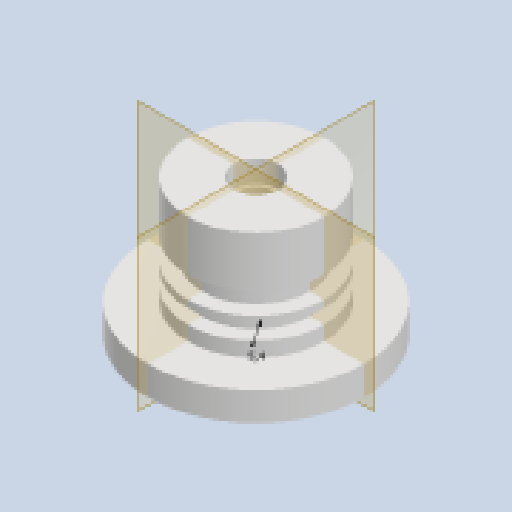
# Autodesk Inventor part: диск
Saved by Autodesk Inventor 2024.2 (Build 282272000, 272)
## iProperties
Created: 2025-11-25
Part Number: диск
Material: Типовые
Document SubType Name: Modeling
Designer: katya_notebook
Density: 1 g/cm^3
Appearance: По умолчанию
Author: katya_notebook
Autodesk Inventor part; units mm, degrees
ref_plane "XZ Plane" through (0, 0, 0) normal (0, 1, 0) x (-1, 0, 0)
sketch "Эскиз1" plane through (0, 0, 0) normal (0, 1, 0) x (-1, 0, 0)
  circle A0 centre (0, 0) radius 9.5
  dimension "d0" = 19
  constraints: 1 centre point, 1 coincident
  measures "d0" diameter of A0
extrude "Выдавливание1" add sketch "Эскиз1" along normal blind 5
sketch "Эскиз2" plane through (0, 0, 0) normal (0, -1, 0) x (1, 0, 0)
  circle A0 centre (0, 0) radius 7.5
  dimension "d3" = 15
  constraints: 1 centre point, 1 coincident
  measures "d3" diameter of A0
extrude "Выдавливание2" add sketch "Эскиз2" along normal blind 3
sketch "Эскиз3" plane through (0, -3, 0) normal (0, -1, 0) x (1, 0, 0)
  circle A0 centre (0, 0) radius 9.5
  dimension "d15" = 19
  constraints: 1 centre point, 1 coincident
  measures "d15" diameter of A0
extrude "Выдавливание3" add sketch "Эскиз3" along normal blind 1
sketch "Эскиз4" plane through (0, -4, 0) normal (0, -1, 0) x (1, 0, 0)
  circle A0 centre (0, 0) radius 7.5
  dimension "d17" = 15
  constraints: 1 centre point, 1 coincident
  measures "d17" diameter of A0
extrude "Выдавливание4" add sketch "Эскиз4" along normal blind 2
sketch "Эскиз5" plane through (0, -6, 0) normal (0, -1, 0) x (1, 0, 0)
  circle A0 centre (0, 0) radius 9.5
  dimension "d16" = 19
  constraints: 1 centre point, 1 coincident
  measures "d16" diameter of A0
extrude "Выдавливание5" add sketch "Эскиз5" along normal blind 2
sketch "Эскиз8" plane through (0, -8, 0) normal (0, -1, 0) x (1, 0, 0)
  circle A0 centre (0, 0) radius 15
  dimension "d21" = 30
  constraints: 1 centre point, 1 coincident
  measures "d21" diameter of A0
extrude "Выдавливание8" add sketch "Эскиз8" along normal blind 2
sketch "Эскиз6" plane through (0, 5, 0) normal (0, 1, 0) x (1, 0, 0)
  circle A0 centre (0, 0) radius 2.6
  dimension "d12" = 5.2
  constraints: 1 centre point, 1 coincident
  measures "d12" diameter of A0
extrude "Выдавливание6" cut sketch "Эскиз6" against normal blind 27
sketch "Эскиз10" plane through (0, -10, 0) normal (0, -1, 0) x (1, 0, 0)
  circle A0 centre (0, 0) radius 15 projected
  circle A1 centre (0, 0) radius 15
  circle A2 centre (0, 0) radius 2.5 projected
  circle A3 centre (0, 0) radius 2.5
  constraints: 2 centre point, 2 coincident, 2 concentric
ref_plane "РабПлоскость1" through (-11.6426, -12, -11.6426) normal (0, -1, 0) x (1, 0, 0)
extrude "Выдавливание10" add sketch "Эскиз10" along normal up to surface (2 mm away)
sketch "Эскиз11" plane through (0, -12, 0) normal (0, -1, 0) x (1, 0, 0)
  circle A0 centre (0, 0) radius 5 projected
  circle A1 centre (0, 0) radius 5
  circle A2 centre (0, 0) radius 2.7
  point P0 (0, 0)
  dimension "d38" = 5.4
  constraints: 2 centre point, 1 concentric
  measures "d38" diameter of A2
ref_plane "РабПлоскость2" through (-5.2921, -22, -5.2921) normal (0, -1, 0) x (1, 0, 0)
sketch "Эскиз13" plane through (0, 5, 0) normal (0, 1, 0) x (1, 0, 0)
  circle A0 centre (0, 0) radius 9.5
  constraints: 1 centre point, 1 coincident
ref_plane "РабПлоскость3" through (-15.9179, 7, -15.9179) normal (0, 1, 0) x (0.0631907, 0, 0.9980015)
extrude "Выдавливание14" add sketch "Эскиз13" along normal up to surface (2 mm away)
sketch "Эскиз14" plane through (0, 7, 0) normal (0, 1, 0) x (1, 0, 0)
  circle A0 centre (0, 0) radius 3.1
  dimension "d48" = 6.2
  constraints: 1 centre point, 1 coincident
  measures "d48" diameter of A0
extrude "Выдавливание15" cut sketch "Эскиз14" against normal blind 3
